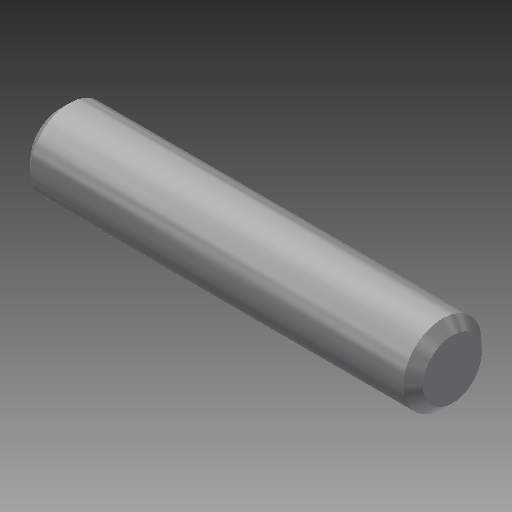
# Autodesk Inventor part: Eje motor - Interno
Saved by Autodesk Inventor 2019 (Build 230136000, 136)
## iProperties
Created: 2019-11-15
Part Number: Eje motor - Interno
Material: Steel
Document SubType Name: Modeling
Designer: Domenico
Density: 1 g/cm^3
Appearance: Steel
CustomPartVersion: 1
Author: Domenico
Autodesk Inventor part; units mm, degrees
ref_plane "Start Plane" through (0, 0, 0) normal (1, 0, 0) x (0, 1, 0)
ref_plane "XZ Plane" through (0, 0, 0) normal (0, 1, 0) x (-1, 0, 0)
ref_plane "XY Plane" through (0, 0, 0) normal (0, 0, 1) x (1, 0, 0)
sketch "Main Sketch" plane through (0, 0, 0) normal (0, 0, 1) x (1, 0, 0)
  line L0 (0, 0) -> (20, 0)
  line L1 (0, 0) -> (0, 2)
  line L2 (20, 2) -> (20, 0)
  line L3 (0, 2) -> (20, 2)
  dimension "d3" = 4
  constraints: 8 end point, 3 horizontal, 2 vertical
  measures "d3" diameter of L3 L0
revolve "Revolution1" add sketch "Main Sketch" angle 360 about axis through (0, 0, 0) along (1, 0, 0)
chamfer "Chamfer1" distance 0.5 angle 45 1 edges at (0, -2, 0) measured on face at (13.3333, 1.9741, -0.3208)
chamfer "Chamfer2" distance 0.5 angle 45 1 edges at (20, -2, 0) measured on face at (13.5, 1.9935, -0.1609)
body "Solid1"
